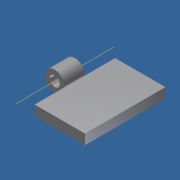
# Autodesk Inventor part: hinge one prong
Saved by Autodesk Inventor 2012 (Build 160160000, 160)
## iProperties
Created: 2012-02-06
Part Number: hinge one prong
Material: Default
Document SubType Name: Modeling
Designer: Allison Garza
Density: 1 g/cm^3
Author: Allison Garza
Autodesk Inventor part; units mm, degrees
ref_plane "YZ Plane" through (0, 0, 0) normal (1, 0, 0) x (0, 1, 0)
ref_plane "XZ Plane" through (0, 0, 0) normal (0, 1, 0) x (-1, 0, 0)
ref_plane "XY Plane" through (0, 0, 0) normal (0, 0, 1) x (1, 0, 0)
sketch "Sketch1" plane through (0, 0, 0) normal (0, 0, 1) x (1, 0, 0)
  circle A0 centre (0, 0) radius 3.175
  circle A1 centre (0, 0) radius 1.5875
  line L0 (0, -3.175) -> (19.05, -3.175)
  line L1 (19.05, -3.175) -> (19.05, 0)
  line L2 (19.05, 0) -> (1.5875, 0)
  line L3 (0, -1.5875) -> (0, -3.175)
  dimension "d1" = 6.35
  dimension "d0" = 3.175
  dimension "d2" = 3.175
  dimension "d3" = 19.05
  constraints: 8 end point, 2 coincident, 2 parallel, 2 point on circle, 1 centre point, 1 horizontal, 1 perpendicular, 1 vertical alignment, 2 other
  measures "d0" diameter of A1
  measures "d2" distance of L0.end L1.end
  measures "d3" distance of L0.start L0.end
extrude "Extrusion1" add sketch "Sketch1" along normal blind 25.4 contours L2 A1 L3 A0 | L2 L1 L0 A0 | A0 L3 A1 L2
sketch "Sketch2" plane through (0, -3.175, 0) normal (0, -1, 0) x (1, 0, 0)
  line L0 (19.05, 25.4) -> (0, 25.4) projected
  line L1 (0, 0) -> (19.05, 0) projected
  line L2 (3.175, 9.525) -> (-3.175, 9.525)
  line L3 (-3.175, 9.525) -> (-3.175, 15.875)
  line L4 (-3.175, 15.875) -> (3.175, 15.875)
  line L5 (3.175, 15.875) -> (3.175, 9.525)
  line L6 (-1.5875, 25.4) -> (1.5875, 25.4) projected
  line L7 (-3.175, 9.525) -> (3.175, 9.525)
  line L8 (3.175, 9.525) -> (3.175, 0)
  line L9 (3.175, 0) -> (-3.175, 0)
  line L10 (-3.175, 0) -> (-3.175, 9.525)
  line L11 (-3.175, 15.875) -> (3.175, 15.875)
  line L12 (3.175, 15.875) -> (3.175, 25.4)
  line L13 (3.175, 25.4) -> (-3.175, 25.4)
  line L14 (-3.175, 25.4) -> (-3.175, 15.875)
  line L15 (3.175, 9.525) -> (3.175, 0)
  line L16 (0, 0) -> (3.175, 0)
  dimension "d6" = 6.35
  dimension "d7" = 6.35
  dimension "d8" = 9.525
  dimension "d9" = 3.175
  dimension "d10" = 3.175
  constraints: 28 end point, 6 parallel, 4 perpendicular, 3 horizontal, 2 point on line, 1 collinear
  measures "d6" distance of L3.end L4.end
  measures "d7" distance of L2.end L3.end
  measures "d8" distance from line of L6 L3.end
  measures "d9" horizontal distance of L0.end L4.end
  measures "d10" distance of L8.end L1.start
extrude "Extrusion2" cut sketch "Sketch2" against normal blind 25.4 contours L12 L4 L14 L13 L6 L0 | L8 L1 L9 L10 L2
body "Solid1"
